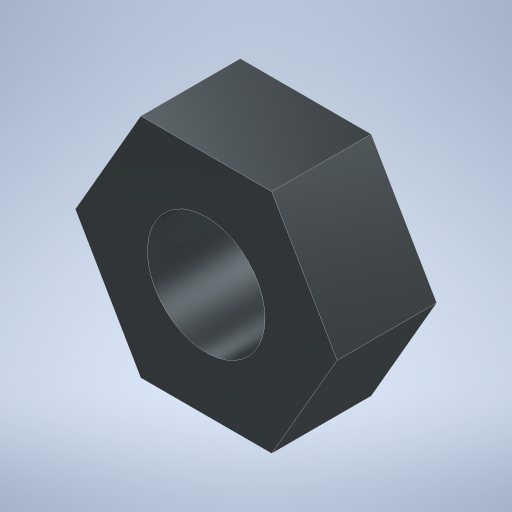
# Autodesk Inventor part: fasten_nut
Saved by Autodesk Inventor 2023 (Build 270158000, 158)
## iProperties
Created: 2023-03-26
Part Number: fasten_nut
Material: Iron, Cast
Document SubType Name: Modeling
Designer: maste
Density: 7.15 g/cm^3
Appearance: Iron Gray
Author: maste
Autodesk Inventor part; units mm, degrees
ref_plane "YZ Plane" through (0, 0, 0) normal (1, 0, 0) x (0, 1, 0)
ref_plane "XZ Plane" through (0, 0, 0) normal (0, 1, 0) x (-1, 0, 0)
ref_plane "XY Plane" through (0, 0, 0) normal (0, 0, 1) x (1, 0, 0)
sketch "Sketch1" plane through (0, 0, 0) normal (0, 0, 1) x (1, 0, 0)
  line L0 (1.5588, 2.7) -> (3.1177, 0)
  line L1 (3.1177, 0) -> (1.5588, -2.7)
  line L2 (1.5588, -2.7) -> (-1.5588, -2.7)
  line L3 (-1.5588, -2.7) -> (-3.1177, 0)
  line L4 (-3.1177, 0) -> (-1.5588, 2.7)
  line L5 (-1.5588, 2.7) -> (1.5588, 2.7)
  circle A0 centre (0, 0) radius 1.4
  dimension "d0" = 5.4
  dimension "d1" = 2.8
  constraints: 12 end point, 2 coincident, 1 centre point, 13 other
  measures "d0" distance between parallel lines of L2 L5
  measures "d1" diameter of A0
extrude "Extrusion1" add sketch "Sketch1" along normal blind 2.37
body "Solid1"
